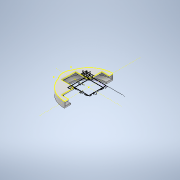
# Autodesk Inventor part: Cycloid_1_v1
Saved by Autodesk Inventor 2020.3 (Build 243373000, 373)
## iProperties
Created: 2021-04-14
Part Number: Cycloid_1_v1
Material: Generic
Document SubType Name: Modeling
Designer: sanyi
Density: 1 g/cm^3
Appearance: Default
Author: sanyi
Autodesk Inventor part; units mm, degrees
ref_plane "YZ Plane" through (0, 0, 0) normal (1, 0, 0) x (0, 1, 0)
ref_plane "XZ Plane" through (0, 0, 0) normal (0, 1, 0) x (-1, 0, 0)
ref_plane "XY Plane" through (0, 0, 0) normal (0, 0, 1) x (1, 0, 0)
sketch "Sketch1" plane through (0, 0, 0) normal (0, 1, 0) x (-1, 0, 0)
  circle A0 centre (0, 0) radius 65.1
  line L0 (0, 138.8733) -> (0, -146.6954) construction
  line L1 (93.3306, 0) -> (-93.3306, 0) construction
  circle A1 centre (0, 0) radius 68.1
  line L2 (57.1, 20) -> (57.1, -20)
  line L3 (20, -57.1) -> (-20, -57.1)
  line L4 (-20, 57.1) -> (20, 57.1)
  line L5 (65.1, 65.1) -> (65.1, -65.1) construction
  line L6 (65.1, -65.1) -> (-65.1, -65.1) construction
  line L7 (-65.1, -65.1) -> (-65.1, 65.1) construction
  line L8 (-65.1, 65.1) -> (65.1, 65.1) construction
  line L9 (20, 57.1) -> (20, 20)
  line L10 (20, 20) -> (57.1, 20)
  line L11 (57.1, -20) -> (20, -20)
  line L12 (20, -20) -> (20, -57.1)
  line L13 (-10, 57.1) -> (-10, 64.3274)
  line L14 (10, 57.1) -> (10, 64.3274)
  line L15 (0, 65.1) -> (0, 68.1)
  line L16 (-10, -57.1) -> (-10, -64.3274)
  line L17 (10, -57.1) -> (10, -64.3274)
  line L18 (0, -65.1) -> (0, -68.1)
  arc A2 (65.1, -19.99) -> (65.1, 19.99) centre (38.6291, 0) ccw
  line L19 (68.1, -28.2646) -> (68.1, 27.9977) construction
  line L20 (71.8, 26.7554) -> (71.8, -21.8254) construction
  line L21 (0, -65.1) -> (0, -57.1)
  line L22 (0, 57.1) -> (0, 65.1)
  dimension "d0" = 130.2
  dimension "d1" = 3
  dimension "d2" = 8
  dimension "d3" = 8
  dimension "d4" = 8
  dimension "d5" = 40
  dimension "d6" = 40
  dimension "d7" = 40
  dimension "d32" = 3.7
  constraints: 46 end point, 13 perpendicular, 9 symmetric about line, 7 point on circle, 6 point on line, 5 midpoint, 4 tangent, 3 centre point, 2 coincident, 2 parallel, 1 collinear, 1 horizontal, 1 vertical, 4 other
  measures "d0" diameter of A0
  measures "d1" radial gap between concentric circles of A1 A0
  measures "d2" distance between parallel lines of L2 L5
  measures "d3" distance between parallel lines of L4 L8
  measures "d4" distance between parallel lines of L6 L3
  measures "d5" distance of L2.start L2.end
  measures "d6" distance of L3.start L3.end
  measures "d7" distance of L4.start L4.end
  measures "d32" distance between parallel lines of L19 L20
extrude "Extrusion1" add sketch "Sketch1" along normal blind 5 contours A0 L17 L3 L12 L11 L2 L10 L9 L4 L14 | A0 L15 A1 L18 | L14 L4 L22 A0 | A0 L21 L3 L17 | A2 A1 picked at (65.7199, -5.652)
extrude "Extrusion3" add sketch "Sketch1" against normal blind 8.1 contours A0 L15 A1 L18 | A2 A1 picked at (65.7199, -5.652)
sketch "Sketch2" plane through (0, -8.1, 0) normal (0, -1, 0) x (1, 0, 0)
  circle A0 centre (0, 0) radius 65.1 projected
  circle A1 centre (0, 0) radius 68.1 projected
  arc A2 (-65.1, 19.99) -> (-65.1, -19.99) centre (-38.6291, 0) ccw projected
  line L0 (0, 65.1) -> (0, 68.1) projected
  line L1 (0, -68.1) -> (0, -65.1) projected
  line L2 (0, 138.8733) -> (0, -146.6954) construction
  line L3 (-93.3306, 0) -> (93.3306, 0) construction
  circle A3 centre (0, 0) radius 50.1
  line L4 (-4, -64.977) -> (-4, -49.9401)
  line L5 (0, -50.1) -> (0, -65.1)
  line L6 (-4, -64.977) -> (-4, -67.9824)
  arc A4 (-65.1, -19.99) -> (0, -68.1) centre (0, 0) ccw projected
  line L7 (-4, 64.977) -> (-4, 49.9401)
  line L8 (0, 50.1) -> (0, 65.1)
  line L9 (-4, 64.977) -> (-4, 67.9824)
  dimension "d14" = 15
  dimension "d15" = 4
  constraints: 12 end point, 5 point on circle, 5 symmetric about line, 1 centre point, 1 coincident, 1 collinear, 1 vertical, 3 other
  measures "d14" radial gap between concentric circles of A0 A3
  measures "d15" distance of the line from the sketch origin of L4
extrude "Extrusion4" add sketch "Sketch2" along normal blind 4 contours L8 A3 L7 A0 | A0 L9 A1 L0 | L1 A1 L6 A0 | A0 L4 A3 L5 | L7 A3 L4 A0 | A0 L6 A1 L9 | A1 A2
fillet "Fillet5" radius 1 14 edges at (-50.1, -8.1, 0) (0, -8.1, 57.6) (0, -8.1, -57.6) (-20, 0, 38.55) (-10, 0, 57.1) (0, 0, 61.1) (-38.55, 0, 20) (-57.1, 0, 0) (-38.55, 0, -20) (-20, 0, -38.55) (-10, 0, -57.1) (0, 0, -61.1) (0, -4.05, 65.1) (0, -4.05, -65.1)
fillet "Fillet6" radius 3 4 edges at (-20.2929, 0.2929, 20.2929) (-20, 3, 20) (-20.2929, 0.2929, -20.2929) (-20, 3, -20)
fillet "Fillet7" radius 10 2 edges at (-65.1, -3.55, 19.99) (-65.1, -3.55, -19.99)
sketch "Sketch4" plane through (0, 5, 0) normal (0, 1, 0) x (1, 0, 0)
  line L0 (20, -20) -> (-20, -20)
  line L1 (-20, -20) -> (-20, 20)
  line L2 (-20, 20) -> (20, 20)
  line L3 (20, 20) -> (20, -20)
  line L4 (0, -138.8733) -> (0, 146.6954) construction
  line L5 (-93.3306, 0) -> (93.3306, 0) construction
  line L6 (-20.1, 20.1) -> (20, 20.1)
  line L7 (20, 20.1) -> (20, 29.1)
  line L8 (20, 29.1) -> (-20.1, 29.1)
  line L9 (-29.1, 29.1) -> (-29.1, 21.9) construction
  line L10 (-29.1, -20) -> (-20.1, -20)
  line L11 (-20.1, -20) -> (-20.1, 20.1)
  line L12 (-20.1, 20.1) -> (-20.1, 29.1)
  line L13 (-20.1, 35.5) -> (-43.6, 35.5)
  line L14 (-43.6, 35.5) -> (-43.6, 21.9)
  line L15 (-43.6, 21.9) -> (-20.1, 21.9)
  line L16 (-27.1, 32) -> (-27.1, 26.2)
  line L17 (-27.1, 26.2) -> (-40.1, 26.2)
  line L18 (-40.1, 26.2) -> (-40.1, 32)
  line L19 (-40.1, 32) -> (-27.1, 32)
  line L20 (27.1735, 25.9682) -> (-9.4534, 25.9682) construction
  line L21 (75.2022, 29.1) -> (26.3609, 29.1) construction
  line L22 (-29.1, 21.9) -> (-29.1, -20)
  line L23 (-20.1, 29.1) -> (-29.1, 29.1) construction
  line L24 (-29.1, 21.9) -> (-29.1, 20.1)
  arc A0 (-20.1, 29.1) -> (-29.1, 20.1) centre (-20.1, 20.1) ccw construction
  line L25 (-21.9, 21.9) -> (-21.9, 35.5) construction
  line L26 (-20.1, 35.5) -> (-20.1, 29.1)
  arc A1 (-27.3, 21.9) -> (-20.1, 29.1) centre (-27.3, 29.1) ccw
  line L27 (-20.1, -20) -> (-20.1, -30)
  line L28 (-20.1, -30) -> (-29.1, -30)
  line L29 (-29.1, -30) -> (-29.1, -20)
  arc A2 (-23, 20) -> (-20, 23) centre (-23, 23) ccw projected
  line L30 (-20, 23) -> (-20, 57.1) projected
  line L31 (-20, 57.1) -> (0, 57.1) projected
  line L32 (0, 57.1) -> (0, 68.1) projected
  arc A3 (0, 68.1) -> (-64.6489, 21.4039) centre (0, 0) ccw projected
  arc A4 (-65.916, 18.8609) -> (-64.6489, 21.4039) centre (-74.1422, 24.5469) ccw projected
  arc A5 (-65.916, 18.8609) -> (-65.916, -18.8609) centre (-38.6291, 0) ccw projected
  arc A6 (-64.6489, -21.4039) -> (-65.916, -18.8609) centre (-74.1422, -24.5469) ccw projected
  arc A7 (-64.6489, -21.4039) -> (0, -68.1) centre (0, 0) ccw projected
  line L33 (0, -68.1) -> (0, -57.1) projected
  line L34 (0, -57.1) -> (-20, -57.1) projected
  line L35 (-20, -57.1) -> (-20, -23) projected
  arc A8 (-20, -23) -> (-23, -20) centre (-23, -23) ccw projected
  line L36 (-23, -20) -> (-57.1, -20) projected
  line L37 (-57.1, -20) -> (-57.1, 20) projected
  line L38 (-57.1, 20) -> (-23, 20) projected
  line L39 (-20.1, -30) -> (-20, -30)
  dimension "d36" = 40
  dimension "d37" = 40
  dimension "d39" = 9
  dimension "d40" = 5.8
  dimension "d41" = 13
  dimension "d42" = 9
  dimension "d43" = 4.3
  dimension "d44" = 7
  dimension "d45" = 3.5
  dimension "d46" = 1.8
  dimension "d47" = 3.5
  dimension "d48" = 0.1
  dimension "d49" = 10
  constraints: 58 end point, 18 perpendicular, 12 point on line, 8 parallel, 4 point on circle, 3 collinear, 3 tangent, 2 centre point, 1 horizontal, 3 other
  measures "d36" distance of L0.start L0.end
  measures "d37" distance of L2.end L0.start
  measures "d39" distance of L6.end L7.end
  measures "d40" distance of L18.end L17.end
  measures "d41" distance of L17.end L17.start
  measures "d42" distance between parallel lines of L6 L21
  measures "d43" distance between parallel lines of L15 L17
  measures "d44" distance between parallel lines of L11 L16
  measures "d45" distance between parallel lines of L13 L19
  measures "d46" distance between parallel lines of L12 L25
  measures "d47" distance between parallel lines of L14 L18
  measures "d48" distance between parallel lines of L1 L11
  measures "d49" distance between parallel lines of L10 L28
body "Solid1"
